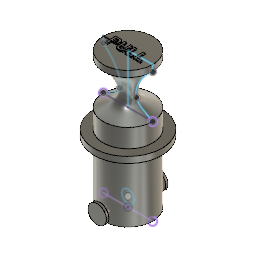
pull knob v7 (Autodesk Fusion 360 design; units mm, degrees)
Autodesk Fusion 360 part; units mm, degrees
sketch "Sketch1" plane through (0, 0, 0) normal (0, 0, 1) x (1, 0, 0)
  circle A0 centre (0, 0) radius 20
  dimension "d1" = 40
  constraint coincident A0.centre origin
  measures "d1" diameter of A0
extrude "Extrude1" add sketch "Sketch1" along normal blind 70 makes body 1
sketch "Sketch2" plane through (0, 0, 0) normal (0, 1, 0) x (1, 0, 0)
  circle A0 centre (0, -7.5) radius 5
  spline S0 degree 5 poles (-20.0003, -70) (-19.0832, -70.5108) (-17.302, -71.4894) (-14.7896, -72.828) (-11.7883, -74.4194) (-8.7922, -76.4321) (-6.7657, -78.8569) (-5.9072, -82.0081) (-6.3018, -85.9495) (-7.9319, -90.5107) (-10.7466, -95.4152) (-13.9021, -99.3677) (-16.761, -102.235) (-18.8843, -104.0881) (-20.0003, -105) knots 0 0 0 0 0 0 0.1 0.2 0.3 0.4 0.5 0.6 0.7 0.8 0.9 1 1 1 1 1 1
  line L0 (-20.0003, -105) -> (-20.0003, -110)
  line L1 (-20.0003, -110) -> (-0.0003, -110)
  line L2 (-0.0003, -110) -> (-0.0003, -70)
  line L3 (-0.0003, -70) -> (-20.0003, -70)
  line L4 (19.9997, -105) -> (19.9997, -110)
  line L5 (-0.0003, -110) -> (-0.0003, -70)
  spline S1 degree 5 poles (19.9997, -70) (19.0826, -70.5108) (17.3014, -71.4894) (14.789, -72.828) (11.7877, -74.4194) (8.7916, -76.4321) (6.7651, -78.8569) (5.9066, -82.0081) (6.3012, -85.9495) (7.9313, -90.5107) (10.746, -95.4152) (13.9015, -99.3677) (16.7604, -102.235) (18.8837, -104.0881) (19.9997, -105) knots 0 0 0 0 0 0 0.1 0.2 0.3 0.4 0.5 0.6 0.7 0.8 0.9 1 1 1 1 1 1
  line L6 (-24.6739, -67.3968) -> (-15.3267, -72.6032)
  line L7 (-15.7976, -101.5658) -> (-24.2031, -108.4342)
  line L8 (24.6733, -67.3968) -> (15.3261, -72.6032)
  line L9 (15.7969, -101.5658) -> (24.2024, -108.4342)
  line L10 (19.9997, -110) -> (-0.0003, -110)
  line L11 (-0.0003, -70) -> (19.9997, -70)
  line L12 (-20, -70) -> (20, -70)
  line L13 (-20, 0) -> (20, 0)
  point P0 (-6.5881, -80.1815)
  point P1 (6.5875, -80.1815)
  dimension "d4" = 10
  dimension "d5" = 7.5
  dimension "d6" = 35
  dimension "d7" = 5
  dimension "d9" = 20
  dimension "d10" = 20
  constraint vertical L0
  constraint perpendicular L0 L1
  constraint perpendicular L1 L2
  constraint perpendicular L2 L3
  constraint midpoint S0.start L6
  constraint midpoint S0.end L7
  constraint symmetric S0.start L2 S1.start
  constraint symmetric P0 L2 P1
  constraint symmetric S0.end L2 L4.start
  constraint symmetric L0.end L2 L4.end
  constraint symmetric L1.end L2 L5.start
  constraint symmetric L3.start L2 L5.end
  constraint symmetric L2 L6.start L8.start
  constraint symmetric L2 L6.end L8.end
  constraint symmetric L2 L7.start L9.start
  constraint symmetric L2 L7.end L9.end
  constraint collinear L11 L12
  measures "d4" diameter of A0
  measures "d5" distance of origin A0.centre
  measures "d6" distance of S0.start S0.end
  measures "d7" distance of S0.end L0.end
  measures "d9" distance of L0.end L1.end
  measures "d10" distance of S0.start L2.end
revolve "Revolve1" add sketch "Sketch2" angle 360 about axis through (-0.0003, 0, 110) along (0, 0, -1) contours S0 L0 L1 L2 L3 L5 L12 bodies 1
extrude "Extrude2" add sketch "Sketch2" along normal mid plane 50 separate body contours A0 makes body 2
sketch "Sketch3" plane through (0, 0, 110) normal (0, 0, 1) x (-1, 0, 0)
  circle A0 centre (0.0003, 0) radius 20
  line L0 (20.0003, -20) -> (-19.9997, -20)
  line L1 (-19.9997, -20) -> (-19.9997, 20)
  line L2 (-19.9997, 20) -> (20.0003, 20)
  line L3 (20.0003, 20) -> (20.0003, -20)
  line L4 (20.0003, 20) -> (-19.9997, 20) construction
  line L5 (-19.9997, 20) -> (-19.9997, -20) construction
  line L6 (-19.9997, -20) -> (20.0003, -20) construction
  line L7 (20.0003, -20) -> (20.0003, 20) construction
  dimension "d14" = 40
  dimension "d15" = 40
  dimension "d16" = 8
  text T0 "PULL" font "Arial" height 8 bold align centre middle in box 40 x 40 at (20.0003, 20) x (-1, 0) y (0, -1) spacing 1
  constraint horizontal L0
  constraint vertical L1
  constraint horizontal L2
  constraint vertical L3
  constraint tangent A0 L0
  constraint tangent A0 L1
  constraint coincident L1.end
  constraint coincident L0.start
  measures "d14" distance of L1.end L2.end
  measures "d15" distance of L0.end L1.end
extrude "Extrude3" add sketch "Sketch3" along normal blind 1 text T0 bodies 1
sketch "Sketch4" plane through (0, -25, 0) normal (0, -1, 0) x (1, 0, 0)
  circle A0 centre (0, 7.5) radius 5
  circle A1 centre (0, 7.5) radius 7.5
  dimension "d19" = 15
  constraint concentric A0 A1
  measures "d19" diameter of A1
extrude "Extrude4" add sketch "Sketch4" against normal blind 2 bodies 2
sketch "Sketch5" plane through (0, 25, 0) normal (0, 1, 0) x (-1, 0, 0)
  circle A0 centre (0, 7.5) radius 5
  circle A1 centre (0, 7.5) radius 7.5
  dimension "d22" = 15
  constraint concentric A0 A1
  measures "d22" diameter of A1
extrude "Extrude5" add sketch "Sketch5" against normal blind 2 bodies 2
ref_plane "WorkPlane1" through (0, 0, 65) normal (0, 0, 1) x (1, 0, 0)
sketch "Sketch6" plane through (0, 0, 65) normal (0, 0, 1) x (1, 0, 0)
  circle A0 centre (0, 0) radius 27.5
  dimension "d34" = 55
  constraint coincident A0.centre origin
  measures "d34" diameter of A0
extrude "Extrude6" add sketch "Sketch6" against normal blind 20 bodies 1
extrude "Extrude7" cut 1 faces at (24.8232, -2.3598, 65) along direction (0, 0, -1) blind 15 on bodies 1 bodies 1
extrude "Extrude8" add 1 faces at (24.8232, -2.3598, 50) along direction (0, 0, 1) blind 5 on bodies 1 bodies 1
extrude "Extrude9" cut 1 faces at (24.8232, -2.3598, 45) along direction (0, 0, 1) blind 5 on bodies 1 bodies 1
